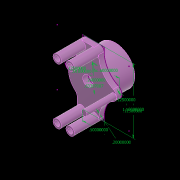
# Autodesk Inventor part: MotorMountShufflerPod
Saved by Autodesk Inventor 2022 (Build 260153000, 153)
## iProperties
Created: 2022-03-05
Part Number: MotorMountShufflerPod
Material: Custom TPU
Document SubType Name: Modeling
Designer: tandu
Density: 1.21 g/cm^3
Appearance: Smooth - Purple
TopStandoffOffset: 0.60000000 in
Author: tandu
Autodesk Inventor part; units mm, degrees
ref_plane "YZ Plane" through (0, 0, 0) normal (1, 0, 0) x (0, 1, 0)
ref_plane "XZ Plane" through (0, 0, 0) normal (0, 1, 0) x (-1, 0, 0)
ref_plane "XY Plane" through (0, 0, 0) normal (0, 0, 1) x (1, 0, 0)
sketch "Sketch1" plane through (0, 0, 0) normal (0, 0, 1) x (1, 0, 0)
  circle A0 centre (0, 0) radius 8.04 construction
  circle A1 centre (0, 0) radius 3.048
  circle A2 centre (0, 0) radius 8.294
  circle A3 centre (0, 0) radius 11.469
  line L0 (6.35, 19.05) -> (-6.35, 19.05)
  line L1 (-6.35, 19.05) -> (-6.35, -19.05)
  line L2 (-6.35, -19.05) -> (6.35, -19.05)
  line L3 (6.35, -19.05) -> (6.35, 19.05)
  line L4 (6.35, 19.05) -> (-6.35, -19.05) construction
  line L5 (-6.35, 19.05) -> (6.35, -19.05) construction
  circle A4 centre (15.24, 0) radius 1.5875
  circle A5 centre (3.81, -16.51) radius 2.54
  circle A6 centre (-3.81, -16.51) radius 2.54
  circle A7 centre (3.81, 16.51) radius 2.54
  circle A8 centre (-3.81, 16.51) radius 2.54
  circle A9 centre (-15.24, 0) radius 1.5875
  line L6 (0, 0) -> (-15.24, 0) construction
  line L7 (0, 0) -> (15.24, 0) construction
  arc A10 (14.8126, -3.175) -> (14.8126, 3.175) centre (13.3185, 0) ccw
  arc A11 (14.8126, -3.175) -> (6.35, -16.51) centre (21.0877, -16.51) ccw
  arc A12 (6.35, 16.51) -> (14.8126, 3.175) centre (21.0877, 16.51) ccw
  line L8 (0, -19.05) -> (0, 19.05) construction
  arc A13 (-14.8126, 3.175) -> (-14.8126, -3.175) centre (-13.3185, 0) ccw
  arc A14 (-6.35, -16.51) -> (-14.8126, -3.175) centre (-21.0877, -16.51) ccw
  arc A15 (-14.8126, 3.175) -> (-6.35, 16.51) centre (-21.0877, 16.51) ccw
  point P0 (-6.35, 9.5507)
  point P1 (6.35, 9.5507)
  point P2 (6.35, -9.5507)
  point P3 (-6.35, -9.5507)
  point P4 (-6.35, -16.51)
  point P5 (-3.81, -19.05)
  point P6 (3.81, -19.05)
  point P7 (6.35, -16.51)
  point P8 (6.35, 16.51)
  point P9 (3.81, 19.05)
  point P10 (-3.81, 19.05)
  point P11 (-6.35, 16.51)
  point P12 (-10.4708, -4.6798)
  point P13 (-15.24, -1.5875)
  point P14 (-15.24, 1.5875)
  point P15 (-10.4708, 4.6798)
  point P16 (15.24, 1.5875)
  point P17 (15.24, -1.5875)
  point P18 (-6.35, 16.51)
  point P19 (-16.8275, 0)
  point P20 (-6.35, -16.51)
  point P21 (16.8275, 0)
  dimension "d0" = 16.08
  dimension "d1" = 6.096
  dimension "d2" = 0.254
  dimension "d3" = 3.175
  dimension "d6" = 12.7
  dimension "d7" = 38.1
  dimension "d10" = 3.175
  dimension "d11" = 5.08
  dimension "d15" = 15.24
  dimension "d19" = 3.175
  constraints: 18 end point, 18 point on circle, 16 centre point, 14 tangent, 7 symmetric about line, 5 midpoint, 4 equal radius, 3 horizontal, 2 coincident, 2 horizontal alignment, 2 parallel, 2 point on line, 1 collinear, 1 perpendicular, 1 vertical alignment, 3 other
  measures "d0" diameter of A0
  measures "d1" diameter of A1
  measures "d2" radial gap between concentric circles of A0 A2
  measures "d3" radial gap between concentric circles of A2 A3
  measures "d6" distance of L2.end L1.end
  measures "d7" distance of L1.end L0.end
  measures "d10" diameter of A4
  measures "d11" diameter of A5
  measures "d15" distance of L6.start L7.end
  measures "d19" vertical distance of L7.end A10.start
extrude "CircularMotorMount" add sketch "Sketch1" against normal blind 13 contours A2 L3 A3 | A2 L1 A3 L3 | L3 A3 L1 A2 | A2 L1 A3
extrude "Plate" add sketch "Sketch1" along normal blind 3.175 contours A2 L3 | A2 L3 A3 | L3 A2 L1 | A2 L1 A3 L3 | L3 A3 L1 A2 | L1 A2 | A2 L1 A3 | A4 | L3 A12 A10 A11 A3 | A3 L1 A8 L0 A7 L3 | L3 A5 L2 A6 L1 A3 | A7 | A5 | A8 | A6
extrude "StandOffLikeThings" add sketch "Sketch1" along normal blind 14.224 from surface at 3.175 contours A4 | A7 | A5 | A8 | A6
fillet "Fillet1" radius 3.175 2 edges at (-6.35, 9.5507, 1.5875) (-6.35, -9.5507, 1.5875)
sketch "Sketch2" plane through (-3.81, 16.51, 17.399) normal (0, 0, 1) x (1, 0, 0)
  circle A0 centre (0, 0) radius 2.54 projected
  circle A1 centre (7.62, 0) radius 2.54 projected
  circle A2 centre (0, -33.02) radius 2.54 projected
  circle A3 centre (7.62, -33.02) radius 2.54 projected
  circle A4 centre (0, -33.02) radius 1.4732
  circle A5 centre (7.62, -33.02) radius 1.4732
  circle A6 centre (0, 0) radius 1.4732
  circle A7 centre (7.62, 0) radius 1.4732
  point P0 (3.81, -16.51)
  dimension "d21" = 2.9464
  constraints: 4 centre point, 4 coincident, 3 equal radius
  measures "d21" diameter of A4
extrude "Extrusion4" cut sketch "Sketch2" against normal blind 9.525 contours A4 | A5 | A6 | A7
extrude "Extrusion5" add sketch "Sketch1" along normal blind 3.175 from surface at 17.399 contours A4
equation "\"d15\" = TopStandoffOffset"
equation "\"TopStandoffOffset\" = 15.24"
body "Solid1"
